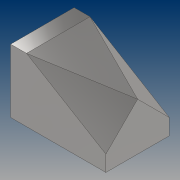
# Autodesk Inventor part: 16
Saved by Autodesk Inventor 2020.2 (Build 242310000, 310)
## iProperties
Created: 2020-09-17
Part Number: 16
Material: 鋼、碳鋼
Document SubType Name: Modeling
Designer: user
Density: 7.85 g/cm^3
Appearance: 半拋光
Mass: 622.767 g
Surface Area: 110.56 cm^2
Volume: 79.3333 cm^3
Author: user
Autodesk Inventor part; units mm, degrees
ref_plane "YZ Plane" through (0, 0, 0) normal (1, 0, 0) x (0, 1, 0)
sketch "草圖1" plane through (0, 0, 0) normal (0, 1, 0) x (-1, 0, 0)
  line L0 (0, 0) -> (-60, 0)
  line L1 (-60, 0) -> (-60, 40)
  line L2 (-60, 40) -> (0, 40)
  line L3 (0, 40) -> (0, 0)
  dimension "d0" = 40
  dimension "d1" = 60
  constraints: 8 end point, 2 parallel, 1 horizontal, 1 perpendicular
  measures "d0" distance of L2.end L0.start
  measures "d1" distance of L0.start L0.end
extrude "擠出1" add sketch "草圖1" along normal blind 40
sketch "草圖3" plane through (60, 0, 40) normal (1, 0, 0) x (0, 0, -1)
  line L0 (40, 40) -> (40, 0) projected
  line L1 (40, 0) -> (0, 0) construction
  line L2 (0, 0) -> (0, 40) construction
  line L3 (0, 40) -> (40, 40) construction
  line L4 (40, 40) -> (0, 40) construction
  line L5 (40, 0) -> (40, 40) projected
  line L6 (40, 10) -> (20, 30)
  line L7 (20, 30) -> (40, 40)
  dimension "d14" = 30
  dimension "d15" = 20
  dimension "d16" = 10
  constraints: 4 end point, 1 point on line
  measures "d14" distance from line of L3 L6.start
  measures "d15" distance from line of L0 L6.end
  measures "d16" distance from line of L6.end L3
ref_plane "工作平面2" through (10, 0, 0) normal (-1, 0, 0) x (0, 0, 1)
sketch "草圖7" plane through (10, 0, 0) normal (-1, 0, 0) x (0, 0, 1)
  line L0 (0, 0) -> (0, 40) construction
  line L1 (0, 40) -> (40, 40) construction
  line L2 (40, 40) -> (40, 0) construction
  line L3 (40, 0) -> (0, 0) construction
  constraints: 1 coincident
loft "斷面混成2" cut profiles "草圖3" section 2 point at (10, 40, 0)
ref_plane "工作平面4" through (0, 0, 20) normal (0, 0, 1) x (1, 0, 0)
mirror "鏡射2" about plane through (0, 0, 20) normal (0, 0, 1) of "斷面混成2"
sketch "草圖18" plane through (60, 0, 0) normal (0, 0, -1) x (-1, 0, 0)
  line L0 (60, 40) -> (60, 0) projected
  line L1 (60, 0) -> (0, 0) projected
  line L2 (0, 0) -> (0, 10) projected
  line L3 (0, 10) -> (50, 40) projected
  line L4 (50, 40) -> (60, 40) projected
  line L5 (50, 40) -> (0, 40) projected
  line L6 (60, 40) -> (50, 40) projected
  line L7 (0, 30) -> (50, 40) projected
  line L8 (50, 40) -> (0, 30)
  line L9 (0, 30) -> (0, 40)
  line L10 (50, 40) -> (0, 40) projected
  line L11 (0, 40) -> (50, 40)
  constraints: 6 end point, 2 collinear, 1 perpendicular
extrude "擠出2" cut sketch "草圖18" against normal blind 45 contours L7 L9 L5
